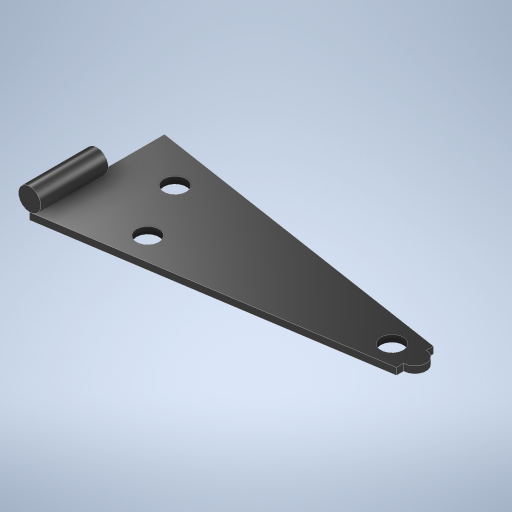
# Autodesk Inventor part: Hinge
Saved by Autodesk Inventor 2024 (Build 280153000, 153)
## iProperties
Created: 2023-06-15
Part Number: Hinge
Material: Generic
Document SubType Name: Modeling
Designer: 18179
Density: 1 g/cm^3
Appearance: Glossy - Black
Author: 18179
Autodesk Inventor part; units mm, degrees
ref_plane "YZ Plane" through (0, 0, 0) normal (1, 0, 0) x (0, 1, 0)
ref_plane "XZ Plane" through (0, 0, 0) normal (0, 1, 0) x (-1, 0, 0)
ref_plane "XY Plane" through (0, 0, 0) normal (0, 0, 1) x (1, 0, 0)
sketch "Sketch1" plane through (0, 0, 0) normal (0, 1, 0) x (-1, 0, 0)
  line L0 (0, 0) -> (73.152, 0)
  line L1 (73.152, 0) -> (73.152, 14.986)
  line L2 (73.152, 14.986) -> (73.152, -14.986)
  circle A0 centre (2.5, 0) radius 2.5
  line L3 (2.5, -2.5) -> (2.5, -4.1002)
  line L4 (2.5, -4.1002) -> (73.152, -14.986)
  line L5 (2.5, 2.5) -> (2.5, 4.1002)
  line L6 (2.5, 4.1002) -> (73.152, 14.986)
  circle A1 centre (7.5955, 0) radius 2.5
  circle A2 centre (62.172, -6.35) radius 2.5
  circle A3 centre (55.5486, 6.35) radius 2.5
  dimension "d3" = 5
  dimension "d0" = 73.152
  dimension "d1" = 14.986
  dimension "d2" = 29.972
  dimension "d4" = 2.5
  dimension "d5" = 1.6002
  dimension "d6" = 5
  dimension "d7" = 5
  dimension "d8" = 5
  dimension "d9" = 6.35
  dimension "d10" = 6.35
  constraints: 14 end point, 3 centre point, 3 point on line, 2 symmetric about line, 1 horizontal, 1 perpendicular, 1 vertical, 3 other
  measures "d0" distance of L0.start L0.end
  measures "d1" distance of L0.end L1.end
  measures "d2" distance of L1.end L2.end
  measures "d4" distance of point (2.5, 0) L0.start
  measures "d5" distance of L3.start L3.end
  measures "d6" diameter of A1
  measures "d7" diameter of A2
  measures "d8" diameter of A3
  measures "d9" distance from line of A2.centre L0
  measures "d10" distance from line of L0 A3.centre
extrude "Extrusion1" add sketch "Sketch1" along normal blind 1.524 contours A0 L0 | L0 A0 | A0 L5 L6 L1 L0 A1 | L0 A1 L2 L4 L3 A0
sketch "Sketch2" plane through (0, 0, 0) normal (0, 0, 1) x (1, 0, 0)
  line L0 (-73.152, 1.524) -> (-2.5, 1.524) projected
  line L1 (-73.152, 1.524) -> (-73.152, 4.024)
  circle A0 centre (-73.152, 4.024) radius 2.5
  point P0 (0, 0)
  dimension "d13" = 2.5
  constraints: 2 end point, 1 coincident, 1 vertical, 1 vertical alignment, 2 other
  measures "d13" distance of L0.start L1.end
extrude "Extrusion2" add sketch "Sketch2" along normal up to surface (14.986 mm away)
body "Solid1"
